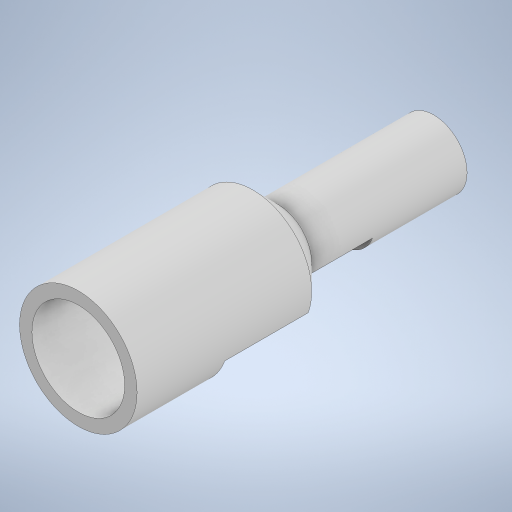
# Autodesk Inventor part: objective
Saved by Autodesk Inventor 2024 (Build 280153000, 153)
## iProperties
Created: 2025-02-23
Part Number: objective
Material: Generic
Document SubType Name: Modeling
Designer: Williamow
Density: 1 g/cm^3
Appearance: Default
Author: Williamow
Autodesk Inventor part; units mm, degrees
ref_plane "YZ Plane" through (0, 0, 0) normal (1, 0, 0) x (0, 1, 0)
ref_plane "XZ Plane" through (0, 0, 0) normal (0, 1, 0) x (-1, 0, 0)
ref_plane "XY Plane" through (0, 0, 0) normal (0, 0, 1) x (1, 0, 0)
sketch "Sketch1" plane through (0, 0, 0) normal (1, 0, 0) x (0, 1, 0)
  line L0 (0, 0) -> (0, 0)
  line L1 (3, 0) -> (3.8, 0)
  line L2 (3.8, 0) -> (3.8, -1.23)
  line L3 (3.8, -1.23) -> (3.8, -8.7)
  line L4 (3.8, -8.7) -> (3.8, -11.3)
  line L5 (3.8, -11.3) -> (3.6318, -11.4682)
  line L6 (2.2, -11.3) -> (3, -10.5)
  line L7 (3, -10.5) -> (3, -9.5)
  line L8 (3, -9.5) -> (2.2, -8.7)
  line L9 (2.2, -8.7) -> (3, -7.9)
  line L10 (3, -5.9) -> (3.8, -5.9)
  line L11 (3.6318, -11.4682) -> (2.159, -12.941)
  line L12 (2.159, -12.941) -> (2.159, -23)
  line L13 (2.159, -23) -> (1.359, -23)
  line L14 (1.359, -23) -> (1.359, -12.141)
  line L15 (1.359, -12.141) -> (2.2, -11.3)
  line L16 (0, 0) -> (0, -2.45)
  line L17 (1.359, -17) -> (2.159, -17)
  line L18 (3, -5.9) -> (3, 0)
  line L19 (3, -5.9) -> (3, -7.9)
  point P0 (3, -10)
  dimension "d1" = 1
  dimension "d3" = 0.8
  dimension "d5" = 3
  dimension "d7" = 10
  dimension "d10" = 0.8
  dimension "d11" = 13
  dimension "d15" = 135
  dimension "d16" = 2.159
  dimension "d18" = 6
  dimension "d22" = 0.8
  dimension "d23" = 3.8
  dimension "d24" = 0.8
  dimension "d25" = 2
  constraints: 40 end point, 6 perpendicular, 6 vertical, 4 horizontal alignment, 3 collinear, 3 point on line, 2 horizontal, 2 parallel, 1 coincident, 1 midpoint, 1 vertical alignment
  measures "d1" distance of L7.start L8.start
  measures "d3" distance between parallel lines of L4 L7
  measures "d5" horizontal distance of L0.start point (3, -10)
  measures "d7" vertical distance of L0.start point (3, -10)
  measures "d10" distance of L12.end L13.end
  measures "d11" vertical distance of L13.end point (3, -10)
  measures "d15" angle of L11 L12
  measures "d16" distance from line of point (0, 0) L12
  measures "d18" distance of L12.end L17.end
  measures "d22" distance of L1.start L2.start
  measures "d23" distance of point (0, 0) L2.start
  measures "d24" horizontal distance of L8.end L8.start
  measures "d25" distance of L10.start L9.end
revolve "Revolution1" add sketch "Sketch1" angle 220 mid plane about axis through (0, 0, 0) along (0, 0, -1)
revolve "Revolution2" add sketch "Sketch1" angle 360 about axis through (0, 0, 0) along (0, 0, -1) contours L1 L2 L3 L10 L18 | L12 L13 L14 L17
body "Solid1"
